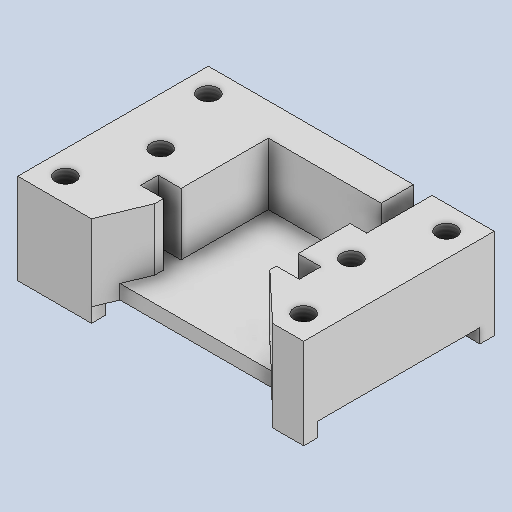
# Autodesk Inventor part: Podstawa
Saved by Autodesk Inventor 2025.2 (Build 292293000, 293)
## iProperties
Created: 2026-05-04
Part Number: Podstawa
Material: Ogólny
Document SubType Name: Modeling
Designer: muszy
Density: 1 g/cm^3
Appearance: Domyślna
Author: muszy
Autodesk Inventor part; units mm, degrees
ref_plane "YZ Plane" through (0, 0, 0) normal (1, 0, 0) x (0, 1, 0)
ref_plane "XZ Plane" through (0, 0, 0) normal (0, 1, 0) x (-1, 0, 0)
ref_plane "XY Plane" through (0, 0, 0) normal (0, 0, 1) x (1, 0, 0)
sketch "Szkic1" plane through (0, 0, 0) normal (0, 1, 0) x (-1, 0, 0)
  line L0 (30, -20) -> (-30, -20)
  line L1 (-30, -20) -> (-30, 20)
  line L2 (-30, 20) -> (30, 20)
  line L3 (30, 20) -> (30, -20)
  line L4 (30, -20) -> (-30, 20) construction
  line L5 (-30, -20) -> (30, 20) construction
  point P0 (0, 0)
  dimension "d0" = 60
  dimension "d1" = 40
  constraints: 12 end point, 2 midpoint, 2 parallel, 1 horizontal, 1 perpendicular
  measures "d0" distance of L0.start L0.end
  measures "d1" distance between parallel lines of L2 L0
extrude "Wyciągnięcie proste1" add sketch "Szkic1" along normal blind 3
sketch "Szkic6" plane through (0, 3, 0) normal (0, 1, 0) x (1, 0, 0)
  line L0 (17.3578, -5.5734) -> (12.5578, -5.5734) projected
  line L1 (12.5578, -5.5734) -> (12.5578, 12.7266) projected
  line L2 (12.5578, 12.7266) -> (-10.1422, 12.7266) projected
  line L3 (-10.1422, -5.5734) -> (-10.1422, 12.7266) projected
  line L4 (-10.1422, -5.5734) -> (-14.9422, -5.5734) projected
  line L5 (-14.9422, -5.5734) -> (-14.9422, -8.2734) projected
  line L6 (-10.1422, -8.2734) -> (-14.9422, -8.2734) projected
  line L7 (-10.1422, -8.2734) -> (-10.1422, -10.0734) projected
  line L8 (-10.1422, -10.0734) -> (12.5578, -10.0734) construction
  line L9 (12.5578, -8.2734) -> (12.5578, -10.0734) projected
  line L10 (17.3578, -8.2734) -> (12.5578, -8.2734) projected
  line L11 (17.3578, -5.5734) -> (17.3578, -8.2734) projected
  line L12 (-8.8922, -2.4734) -> (11.3078, -2.4734) projected
  line L13 (-8.8922, 7.7266) -> (-8.8922, -2.4734) projected
  line L14 (11.3078, 7.7266) -> (-8.8922, 7.7266) projected
  line L15 (11.3078, -2.4734) -> (11.3078, 7.7266) projected
  line L16 (-30, -20) -> (30, -20) projected
  line L17 (30, -20) -> (30, 20) projected
  line L18 (30, -20) -> (30, 20)
  line L19 (-30, 20) -> (-30, -20)
  line L20 (-30, -20) -> (-14.5223, -20)
  line L21 (23.4752, -20) -> (30, -20)
  line L22 (-10.6422, 13.2266) -> (13.0578, 13.2266)
  line L23 (13.4777, 6.2814) -> (13.4777, -4.6535)
  line L24 (13.4777, -4.6535) -> (18.2777, -4.6535)
  line L25 (18.2777, -4.6535) -> (18.2777, -9.1933)
  line L26 (18.2777, -9.1933) -> (13.4777, -9.1933)
  line L27 (13.4777, -9.1933) -> (13.4777, -10.5734)
  line L28 (-10.6422, -10.5734) -> (-10.6422, -8.7734)
  line L29 (-10.6422, -8.7734) -> (-15.4422, -8.7734)
  line L30 (-15.4422, -8.7734) -> (-15.4422, -5.0734)
  line L31 (-15.4422, -5.0734) -> (-10.6422, -5.0734)
  line L32 (-10.6422, -5.0734) -> (-10.6422, 13.2266)
  line L33 (13.4777, -10.5734) -> (23.4752, -20)
  line L34 (-10.6422, -10.5734) -> (-14.5223, -20)
  line L35 (13.4777, 6.2814) -> (16.9504, 6.2814)
  line L36 (16.9504, 6.2814) -> (16.9504, 20)
  line L37 (13.0578, 13.2266) -> (13.0578, 20)
  line L38 (30, 20) -> (16.9504, 20)
  line L39 (13.0578, 20) -> (-30, 20)
  point P0 (0, 0)
  dimension "d4" = 0.5
  constraints: 44 end point, 6 perpendicular, 5 parallel, 3 horizontal, 2 point on line, 7 other
  measures "d4" distance between parallel lines of L3 L32
extrude "Wyciągnięcie proste2" add sketch "Szkic6" along normal blind 13 contours L19 L39 L37 L22 L32 L31 L30 L29 L28 L34 L16 | L33 L27 L26 L25 L24 L23 L35 L36 L38 L17 L16
sketch "Szkic7" plane through (0, 3, 0) normal (0, 1, 0) x (1, 0, 0)
  line L0 (13.0578, 20) -> (13.0578, 13.2266) projected
  line L1 (13.0578, 13.2266) -> (-10.6422, 13.2266) projected
  line L2 (-10.6422, 13.2266) -> (-10.6422, -5.0734) projected
  line L3 (-10.6422, -5.0734) -> (-15.4422, -5.0734) projected
  line L4 (-15.4422, -5.0734) -> (-15.4422, -8.7734) projected
  line L5 (-15.4422, -8.7734) -> (-10.6422, -8.7734) projected
  line L6 (-10.6422, -8.7734) -> (-10.6422, -10.5734) projected
  line L7 (-10.6422, -10.5734) -> (-14.5223, -20) projected
  line L8 (-14.5223, -20) -> (23.4752, -20) projected
  line L9 (23.4752, -20) -> (13.4777, -10.5734) projected
  line L10 (13.4777, -10.5734) -> (13.4777, -9.1933) projected
  line L11 (13.4777, -9.1933) -> (18.2777, -9.1933) projected
  line L12 (18.2777, -9.1933) -> (18.2777, -4.6535) projected
  line L13 (18.2777, -4.6535) -> (13.4777, -4.6535) projected
  line L14 (13.4777, -4.6535) -> (13.4777, 6.2814) projected
  line L15 (13.4777, 6.2814) -> (16.9504, 6.2814) projected
  line L16 (16.9504, 6.2814) -> (16.9504, 20) projected
  line L17 (16.9504, 20) -> (13.0578, 20) projected
  line L18 (1.3504, -15.7734) -> (12.6578, -15.7734) projected
  line L19 (-12.7826, -15.7734) -> (18.9926, -15.7734)
  point P0 (0, 0)
  point P1 (12.6578, -15.7734)
  point P2 (1.3504, -15.7734)
  constraints: 2 end point, 2 point on line, 1 horizontal
extrude "Wyciągnięcie proste3" cut sketch "Szkic7" against normal blind 13 contours L19 L18 L9 L8 L7
sketch "Szkic8" plane through (0, 16, 0) normal (0, 1, 0) x (1, 0, 0)
  line L0 (-30, 20) -> (-30, -20) projected
  line L1 (-30, -20) -> (-14.5223, -20) projected
  line L2 (30, 20) -> (-30, 20) projected
  line L3 (-30, 0) -> (30, 0) construction
  line L4 (0, 20) -> (0, -29.6332) construction
  point P0 (0, 0)
  point P1 (-25, -15)
  point P2 (-25, 15)
  point P3 (25, 15)
  point P4 (25, -15)
  dimension "d9" = 5
  dimension "d10" = 5
  constraints: 4 end point, 3 symmetric about line, 2 midpoint, 1 horizontal, 1 vertical
  measures "d9" distance from line of L0 point (-25, -15)
  measures "d10" distance from line of L1 point (-25, -15)
hole "Otwór1" at (-25, 16, 15) at (-25, 16, -15) at (25, 16, -15) at (25, 16, 15) direction (0, -1, 0) diameter 4.134 depth 5 tip angle 118 thread size "M5x0.8" class "6H" standard "ISO Metric profile"
sketch "Szkic9" plane through (0, 0, 0) normal (0, -1, 0) x (1, 0, 0)
  line L0 (30, 20) -> (30, -20) projected
  line L1 (30, -20) -> (-30, -20)
  line L2 (-30, -20) -> (-30, -17)
  line L3 (-30, -17) -> (30, -17)
  line L4 (30, -17) -> (30, -20)
  line L5 (18.9926, 15.7734) -> (-12.7826, 15.7734) projected
  line L6 (30, 20) -> (23.4752, 20)
  line L7 (23.4752, 17) -> (30, 17)
  line L8 (30, 17) -> (30, 20)
  line L9 (23.4752, 20) -> (18.9926, 15.7734) projected
  line L10 (23.4752, 20) -> (23.4752, 17)
  line L11 (-30, 20) -> (-14.5223, 20) projected
  line L12 (-30, 20) -> (-14.5223, 20)
  line L13 (-14.5223, 17) -> (-30, 17)
  line L14 (-30, 17) -> (-30, 20)
  line L15 (-14.5223, 20) -> (-10.6422, 10.5734) projected
  line L16 (-14.5223, 20) -> (-14.5223, 17)
  point P0 (0, 0)
  dimension "d18" = 60
  dimension "d19" = 3
  dimension "d31" = 3
  dimension "d32" = 3
  constraints: 24 end point, 4 parallel, 3 horizontal, 3 perpendicular, 2 point on line
  measures "d18" distance of L2.end L3.end
  measures "d19" distance between parallel lines of L1 L3
  measures "d31" distance between parallel lines of L13 L11
  measures "d32" distance between parallel lines of L6 L7
extrude "Wyciągnięcie proste4" add sketch "Szkic9" along normal blind 3
sketch "Szkic10" plane through (0, 16, 0) normal (0, 1, 0) x (1, 0, 0)
  line L0 (-30, 20) -> (-30, -20) projected
  line L1 (30, -20) -> (30, 20) projected
  point P0 (0, 0)
  point P1 (-20, 0)
  point P2 (20, 0)
  dimension "d22" = 10
  dimension "d23" = 10
  measures "d22" distance from line of L0 point (-20, 0)
  measures "d23" distance from line of L1 point (20, 0)
hole "Otwór2" at (-20, 16, 0) at (20, 16, 0) direction (0, -1, 0) diameter 4.134 end through all thread size "M5x0.8" class "6H" standard "ISO Metric profile"
